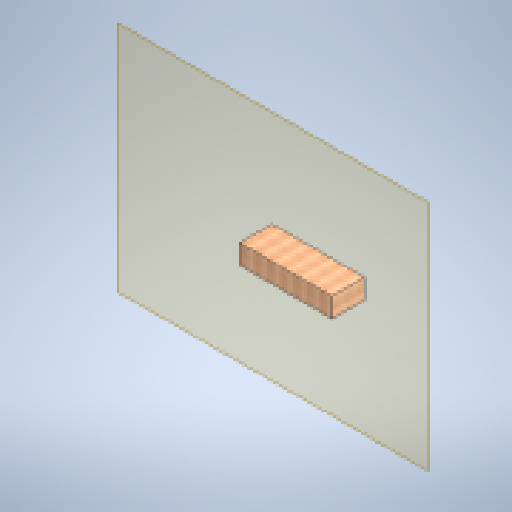
# Autodesk Inventor part: Mueble Tele
Saved by Autodesk Inventor 2024 (Build 280153000, 153)
## iProperties
Created: 2024-04-05
Part Number: Mueble Tele
Material: Genérico
Document SubType Name: Modeling
Designer: sergi
Density: 1 g/cm^3
Appearance: Valor por defecto
Author: sergi
Autodesk Inventor part; units mm, degrees
ref_plane "YZ Plane" through (0, 0, 0) normal (1, 0, 0) x (0, 1, 0)
ref_plane "XZ Plane" through (0, 0, 0) normal (0, 1, 0) x (-1, 0, 0)
ref_plane "XY Plane" through (0, 0, 0) normal (0, 0, 1) x (1, 0, 0)
ref_plane "Plano de trabajo1" through (160.7331, -1577.5, 0) normal (0, 0, 1) x (1, 0, 0)
sketch "Boceto1" plane through (160.7331, -1577.5, 0) normal (0, 0, 1) x (1, 0, 0)
  line L0 (-160.7331, 1577.5) -> (1639.2669, 1577.5)
  line L1 (1639.2669, 1577.5) -> (1639.2669, 1957.5)
  line L2 (1639.2669, 1957.5) -> (-160.7331, 1957.5)
  line L3 (-160.7331, 1957.5) -> (-160.7331, 1577.5)
  dimension "d0" = 1800
  dimension "d1" = 380
  constraints: 8 end point, 2 parallel, 1 horizontal, 1 perpendicular
  measures "d0" distance of L2.end L1.end
  measures "d1" distance of L1.end L0.end
extrude "Extrusión1" add sketch "Boceto1" along normal blind 630
